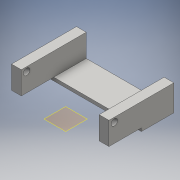
# Autodesk Inventor part: vacuum_cup_base
Saved by Autodesk Inventor 2016 (Build 200138000, 138)
## iProperties
Created: 2016-04-11
Part Number: vacuum_cup_base
Material: 一般
Document SubType Name: Modeling
Designer: Shun Hasegawa
Density: 1 g/cm^3
Appearance: 既定
Author: Shun Hasegawa
Autodesk Inventor part; units mm, degrees
ref_plane "YZ Plane" through (0, 0, 0) normal (1, 0, 0) x (0, 1, 0)
ref_plane "XZ Plane" through (0, 0, 0) normal (0, 1, 0) x (-1, 0, 0)
ref_plane "作業平面1" through (0, 0, -20) normal (0, 0, 1) x (1, 0, 0)
sketch "スケッチ1" plane through (0, 0, -20) normal (0, 0, 1) x (1, 0, 0)
  line L0 (-45, 55) -> (45, 55)
  line L1 (45, 55) -> (45, 25)
  line L2 (45, 25) -> (-45, 25)
  line L3 (-45, 25) -> (-45, 55)
  line L4 (0, 66) -> (0, -11) projected
  line L5 (-63, 0) -> (63, 0) projected
  point P0 (0, 0)
  dimension "d1" = 90
  dimension "d2" = 30
  dimension "d3" = 55
  constraints: 8 end point, 2 parallel, 1 horizontal, 1 perpendicular, 1 other
  measures "d1" distance of L0.start L0.end
  measures "d2" distance of L0.end L1.end
  measures "d3" distance between parallel lines of L5 L0
extrude "押し出し1" add sketch "スケッチ1" along normal blind 3
sketch "スケッチ2" plane through (0, 0, -17) normal (0, 0, 1) x (1, 0, 0)
  line L0 (45, 55) -> (-45, 55) projected
  line L1 (45, 55) -> (36, 55)
  line L2 (36, 55) -> (36, -5)
  line L3 (36, -5) -> (45, -5)
  line L4 (45, -5) -> (45, 55)
  line L5 (-45, 55) -> (-45, 25) projected
  line L6 (-45, 55) -> (-36, 55)
  line L7 (-36, 55) -> (-36, -5)
  line L8 (-36, -5) -> (-45, -5)
  line L9 (-45, -5) -> (-45, 55)
  point P0 (0, 0)
  dimension "d6" = 9
  dimension "d7" = 60
  dimension "d8" = 9
  constraints: 16 end point, 4 parallel, 2 horizontal, 2 perpendicular, 1 point on line
  measures "d6" distance of L2.end L3.end
  measures "d7" distance of L3.end L0.start
  measures "d8" distance of L7.end L8.end
extrude "押し出し2" add sketch "スケッチ2" along normal blind 21
sketch "スケッチ3" plane through (0, 0, 0) normal (1, 0, 0) x (0, 1, 0)
  circle A0 centre (0, 0) radius 3
  dimension "d11" = 6
  constraints: 1 centre point, 1 coincident
  measures "d11" diameter of A0
extrude "押し出し3" cut sketch "スケッチ3" along normal up to surface (90 mm away) from surface at -45
